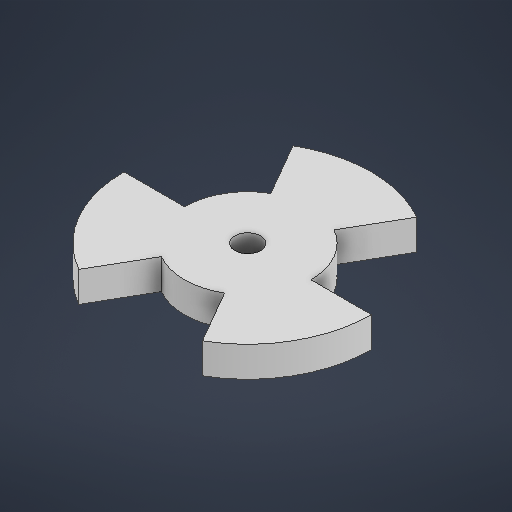
# Autodesk Inventor part: rotor
Saved by Autodesk Inventor 2025.1 (Build 291241020, 241B)
## iProperties
Created: 2024-09-16
Part Number: rotor
Material: Generic
Document SubType Name: Modeling
Designer: maxim
Density: 1 g/cm^3
Appearance: Default
Author: maxim
Autodesk Inventor part; units mm, degrees
ref_plane "YZ Plane" through (0, 0, 0) normal (1, 0, 0) x (0, 1, 0)
ref_plane "XZ Plane" through (0, 0, 0) normal (0, 1, 0) x (-1, 0, 0)
ref_plane "XY Plane" through (0, 0, 0) normal (0, 0, 1) x (1, 0, 0)
sketch "Sketch1" plane through (0, 0, 0) normal (0, 1, 0) x (1, 0, 0)
  circle A0 centre (0, 0) radius 25
  arc A1 (24.4487, 42.3463) -> (-24.4487, 42.3463) centre (0, 0) ccw
  line L0 (12.5, 21.6506) -> (24.4487, 42.3463)
  line L1 (-12.5, 21.6506) -> (-24.4487, 42.3463)
  line L2 (0, 0) -> (0, 84.0286) construction
  line L3 (-12.5, -21.6506) -> (-24.4487, -42.3463)
  arc A2 (-48.8973, 0) -> (-24.4487, -42.3463) centre (0, 0) ccw
  line L4 (-25, 0) -> (-48.8973, 0)
  line L5 (25, 0) -> (48.8973, 0)
  arc A3 (24.4487, -42.3463) -> (48.8973, 0) centre (0, 0) ccw
  line L6 (12.5, -21.6506) -> (24.4487, -42.3463)
  point P0 (25, 0)
  dimension "d0" = 50
  dimension "d1" = 60
  dimension "d2" = 30
  dimension "d5" = 360
  constraints: 14 end point, 8 point on circle, 4 centre point, 2 coincident, 1 vertical, 25 other
  measures "d0" diameter of A0
  measures "d1" angle of L0 L1
  measures "d2" angle of L2 L1
extrude "Extrusion1" add sketch "Sketch1" along normal blind 12
sketch "Sketch4" plane through (0, 0, 0) normal (0, -1, 0) x (1, 0, 0)
  circle A0 centre (0, 0) radius 7.9289 projected
  point P0 (0, 0)
  constraints: 1 coincident
hole "Hole2" at (0, 0, 0) direction (0, 1, 0) diameter 10.2 depth 12
body "Solid1"
